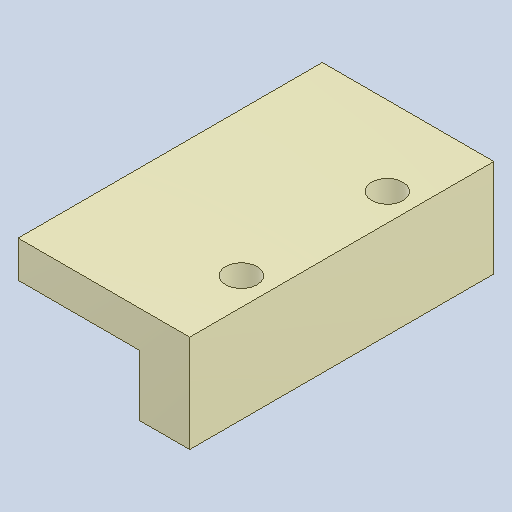
# Autodesk Inventor part: креп_центр_м2
Saved by Autodesk Inventor 2023.1 (Build 271208000, 208)
## iProperties
Created: 2025-12-23
Part Number: креп_центр_м2
Material: Полипропилен
Document SubType Name: Sheet Metal
Designer: DELL
Density: 0.899 g/cm^3
Appearance: Гладкий — пепельный
Sheet Metal Rule: По умолчанию
Author: DELL
Autodesk Inventor part; units mm, degrees
ref_plane "YZ Plane" through (0, 0, 0) normal (1, 0, 0) x (0, 1, 0)
ref_plane "XZ Plane" through (0, 0, 0) normal (0, 1, 0) x (-1, 0, 0)
ref_plane "XY Plane" through (0, 0, 0) normal (0, 0, 1) x (1, 0, 0)
sketch "Эскиз1" plane through (0, 0, 0) normal (0, 0, 1) x (1, 0, 0)
  line L0 (0, 0) -> (-20, 0) construction
  line L1 (-20, 0) -> (-20, 10) construction
  line L2 (-20, 10) -> (0, 10) construction
  line L3 (0, 10) -> (0, 0) construction
  line L4 (-20, 0) -> (8.2, 0) construction
  line L5 (8.2, 0) -> (8.2, 16)
  line L6 (8.2, 16) -> (-20, 16)
  line L7 (-20, 16) -> (-20, 0) construction
  line L8 (-20, 16) -> (-20, 10)
  line L9 (-20, 10) -> (0, 10)
  line L10 (0, 10) -> (0, 0)
  line L11 (0, 0) -> (8.2, 0)
  point P0 (-10, 10)
  dimension "d0" = 20
  dimension "d1" = 10
  dimension "d2" = 6
  dimension "d3" = 8.2
  constraints: 24 end point, 4 parallel, 3 collinear, 3 perpendicular, 2 horizontal, 1 midpoint
  measures "d0" distance of L1.end L2.end
  measures "d1" distance of L0.end L1.end
  measures "d2" distance from line of L6 point (-10, 10)
  measures "d3" distance between parallel lines of L5 L3
extrude "Выдавливание1" add sketch "Эскиз1" along normal blind 50
sketch "Эскиз3" plane through (-20, 16, 0) normal (0, 1, 0) x (1, 0, 0)
  circle A0 centre (23.6882, -13) radius 6 construction
  circle A1 centre (23.6882, -13) radius 2.6
  line L0 (28.2, 0) -> (0, 0) projected
  circle A2 centre (23.6882, -37) radius 2.6
  line L1 (28.2, -50) -> (0, -50) projected
  circle A3 centre (23.6882, -13) radius 9 construction
  circle A4 centre (23.6882, -37) radius 9 construction
  circle A5 centre (23.6882, 52.7109) radius 2.5 construction
  circle A6 centre (23.6882, 52.7109) radius 6
  line L2 (17.6882, 52.7109) -> (17.6882, -70.8519) construction
  line L3 (23.6882, -13) -> (23.6882, -47.2953) construction
  line L4 (20, 0) -> (20, -50) projected
  dimension "d26" = 12
  dimension "d16" = 12
  dimension "d17" = 5.2
  dimension "d20" = 5.2
  dimension "d22" = 24
  dimension "d23" = 18
  dimension "d24" = 18
  dimension "d25" = 13
  constraints: 5 centre point, 4 coincident, 4 end point, 2 vertical, 1 horizontal alignment, 1 parallel, 1 point on line, 1 tangent, 2 other
  measures "d16" diameter of A0
  measures "d17" diameter of A1
  measures "d20" diameter of A2
  measures "d22" distance of A0.centre A2.centre
  measures "d23" diameter of A3
  measures "d24" diameter of A4
  measures "d25" vertical distance of L0.start A0.centre
extrude "Выдавливание4" cut sketch "Эскиз3" against normal blind 20 contours A1 | A2
equation "\"Радиус_гибки\" = Толщина"
equation "\"Ширина_просечки\" = Толщина"
equation "\"Глубина_просечки\" = 0.5 * Толщина"
equation "\"Размер_просечки\" = 4 * Толщина"
equation "\"Мин_остаток\" = 2 * Толщина"
equation "\"Радиус_перехода\" = Радиус_гибки"
equation "\"Радиус_Якоби\" = Радиус_гибки"
equation "\"Размер_зазора\" = Толщина"
equation "\"Толщина\" = 3.048"
